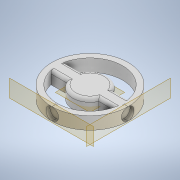
# Autodesk Inventor part: Servo_Kupplung
Saved by Autodesk Inventor 2020 (Build 240168000, 168)
## iProperties
Created: 2020-09-04
Part Number: Servo_Kupplung
Material: Generisch
Document SubType Name: Modeling
Designer: sp
Density: 1 g/cm^3
Appearance: Vorgabe
Author: sp
## iProperties of the stored document _3D-Druck.ipt
Created: 2020-09-04
Part Number: _3D-Druck
Material: Generisch
Document SubType Name: Modeling
Designer: sp
Density: 1 g/cm^3
Appearance: Vorgabe
Author: sp
Autodesk Inventor part; units mm, degrees
ref_plane "XZ Plane" through (0, 0, 0) normal (0, 1, 0) x (-1, 0, 0)
sketch "Skizze1" plane through (0, 0, 0) normal (0, 1, 0) x (-1, 0, 0)
  circle A0 centre (0, 0) radius 24.25
  circle A1 centre (0, 0) radius 20.75
  circle A2 centre (0, 0) radius 3.5
  line L0 (45.7225, 0) -> (-63.662, 0) construction
  line L1 (0, 78.2374) -> (0, -78.2374) construction
  circle A3 centre (15, 0) radius 2
  circle A4 centre (-15, 0) radius 2
  line L2 (0, 3.5) -> (15.1977, 1.9902)
  line L3 (15.1977, -1.9902) -> (0, -3.5)
  line L4 (-14.8023, -1.9902) -> (0, -3.5)
  line L5 (0, 3.5) -> (-15.1977, 1.9902)
  circle A5 centre (0, 0) radius 11
  line L6 (10.0387, 4.4973) -> (20.2568, 4.4973)
  line L7 (-10.0387, 4.4973) -> (-20.2568, 4.4973)
  line L8 (10.0387, -4.4973) -> (20.2568, -4.4973)
  line L9 (-10.0387, -4.4973) -> (-20.2568, -4.4973)
  point P0 (23.8293, 4.4973)
  point P1 (-23.8293, -4.4973)
  point P2 (12.125, -21.0011)
  point P3 (-12.125, 21.0011)
  point P4 (-0.6886, 3.4316)
  point P5 (0.6886, 3.4316)
  point P6 (0.6886, -3.4316)
  point P7 (-0.7066, -3.4279)
  dimension "d0" = 48.5
  dimension "d1" = 41.5
  dimension "d2" = 7
  dimension "d3" = 4
  dimension "d4" = 4
  dimension "d5" = 15
  dimension "d6" = 22
  constraints: 20 end point, 18 point on circle, 9 point on line, 6 centre point, 4 coincident, 3 horizontal, 2 midpoint, 1 parallel, 1 symmetric about line, 1 tangent, 1 vertical
  measures "d0" diameter of A0
  measures "d1" diameter of A1
  measures "d2" diameter of A2
  measures "d3" diameter of A3
  measures "d4" diameter of A4
  measures "d5" distance of point (0, 0) A3.centre
  measures "d6" diameter of A5
ref_plane "Arbeitsebene1" through (0, 3.7, 0) normal (0, 1, 0) x (1, 0, 0)
extrude "Extrusion3" add sketch "Skizze1" along normal blind 8 contours A0 | A1 L8 A5 L3 A3 L2 L6 | L7 A5 L5 A4 L4 L9 A1 | A5 L2 A2 L5 | A5 L4 A2 L3
sketch "Skizze3" plane through (0, 8, 0) normal (0, 1, 0) x (1, 0, 0)
  arc A0 (20.2568, 4.4973) -> (-20.2568, 4.4973) centre (0, 0) ccw projected
  arc A1 (-20.2568, -4.4973) -> (20.2568, -4.4973) centre (0, 0) ccw projected
  line L0 (-20.2568, 4.4973) -> (20.2568, 4.4973)
  line L1 (20.2568, 4.4973) -> (20.2568, -4.4973)
  line L2 (20.2568, -4.4973) -> (-20.2568, -4.4973)
  line L3 (-20.2568, -4.4973) -> (-20.2568, 4.4973)
  constraints: 8 end point, 2 parallel, 1 horizontal, 1 perpendicular, 1 point on circle
extrude "Extrusion4" add sketch "Skizze3" against normal blind 3 contours L1 L2 L3 L0
ref_plane "Arbeitsebene2" through (24.5, 0, 0) normal (1, 0, 0) x (0, 1, 0)
ref_plane "Arbeitsebene3" through (0, 0, 24.5) normal (0, 0, 1) x (1, 0, 0)
sketch "Skizze4" plane through (24.5, 0, 0) normal (1, 0, 0) x (0, 1, 0)
  line L0 (4, 30.052) -> (4, -34.2953) construction
  line L1 (8, -24.25) -> (8, 24.25) construction
  circle A0 centre (4, 0) radius 4
  point P0 (0, 0)
  dimension "d22" = 4
  dimension "d23" = 8
  constraints: 2 end point, 1 centre point, 1 point on line, 1 vertical
  measures "d22" distance between parallel lines of L1 L0
  measures "d23" diameter of A0
sketch "Skizze5" plane through (0, 0, 24.5) normal (0, 0, 1) x (1, 0, 0)
  line L0 (-31.5031, 4) -> (30.733, 4) construction
  line L1 (24.25, 8) -> (-24.25, 8) construction
  circle A0 centre (0, 4) radius 4
  point P0 (0, 0)
  dimension "d24" = 4
  dimension "d25" = 8
  constraints: 2 end point, 1 centre point, 1 horizontal, 1 point on line
  measures "d24" distance between parallel lines of L1 L0
  measures "d25" diameter of A0
extrude "Extrusion5" cut sketch "Skizze4" against normal blind 3
extrude "Extrusion6" cut sketch "Skizze5" against normal blind 3
fillet "Rundung5" radius 2 4 edges at (-15.1477, 8, 4.4973) (-15.1477, 8, -4.4973) (15.1477, 8, 4.4973) (15.1477, 8, -4.4973)
fillet "Rundung6" radius 2 6 edges at (-10.4238, 8, 3.5135) (0, 8, 11) (10.4238, 8, 3.5135) (-10.4238, 8, -3.5135) (0, 8, -11) (10.4238, 8, -3.5135)
